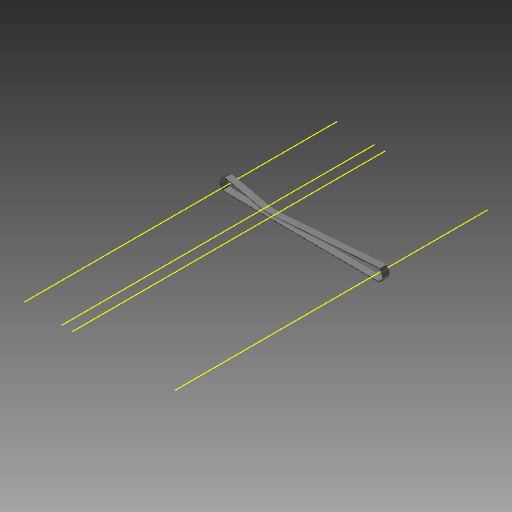
# Autodesk Inventor part: Zahnriemen
Saved by Autodesk Inventor 2019.1 (Build 231200000, 200)
## iProperties
Created: 2018-10-30
Part Number: Zahnriemen
Material: Rubber
Document SubType Name: Modeling
Designer: JochenAlt
Density: 1 g/cm^3
Appearance: Rubber - Black - Version 1.1
CustomPartVersion: 1
Author: JochenAlt
Autodesk Inventor part; units mm, degrees
ref_plane "YZ Plane" through (0, 0, 0) normal (1, 0, 0) x (0, 1, 0)
ref_plane "XZ Plane" through (0, 0, 0) normal (0, 1, 0) x (-1, 0, 0)
ref_plane "XY Plane" through (0, 0, 0) normal (0, 0, 1) x (1, 0, 0)
sketch "Skizzenpfad" plane through (0, 0, 0) normal (0, 0, 1) x (1, 0, 0)
  arc A0 (130.619632, -5.570298) -> (130.240862, 5.554866) centre (130.656885, 0) ccw
  arc A1 (-8.721109, 6.363317) -> (-10.03287, -4.629641) centre (-9.995617, 0.940657) ccw
  arc A2 (24.701763, -1.492183) -> (24.992987, -1.526653) centre (24.999202, -0.226668) ccw
  arc A3 (34.992872, -1.574463) -> (35.096177, -1.570847) centre (34.999088, -0.274478) ccw
  line L0 (35.096177, -1.570847) -> (130.240862, 5.554866)
  line L1 (130.619632, -5.570298) -> (-10.03287, -4.629641)
  line L2 (-8.721109, 6.363317) -> (24.701763, -1.492183)
  line L3 (24.992987, -1.526653) -> (34.992872, -1.574463)
  constraints: 8 end point, 8 point on circle, 4 centre point
ref_plane "Querschnittsebene" through (130.240862, 5.554866, 0) normal (-0.9972072, -0.0746843, 0) x (0, 0, 1)
ref_plane "Arbeitsebene2" through (130.656885, 0, 0) normal (-1, 0, 0) x (0, 0, 1)
ref_plane "Arbeitsebene3" through (-9.995617, 0.940657, 0) normal (0.9456862, -0.3250811, 0) x (0, 0, 1)
sketch "Querschnitt" plane through (130.240862, 5.554866, 0) normal (-0.9972072, -0.0746843, 0) x (0, 0, 1)
  line L0 (-3, 0.3) -> (3, 0.3)
  line L1 (3, 0.3) -> (3, -0.3)
  line L2 (3, -0.3) -> (-3, -0.3)
  line L3 (-3, -0.3) -> (-3, 0.3)
  line L4 (-3, 0) -> (3, 0) construction
  point P0 (0, 0)
  point P1 (0, 0)
  dimension "d0" = 6
  dimension "d4" = 0.3
  dimension "d5" = 0.3
  constraints: 10 end point, 3 midpoint, 2 parallel, 1 coincident, 1 horizontal, 1 perpendicular, 1 other
  measures "d0" distance between parallel lines of L1 L3
  measures "d4" distance between parallel lines of L2 L4
  measures "d5" distance between parallel lines of L4 L0
sweep "Riemen" add profiles "Querschnitt" path "Skizzenpfad" path curves L3 A3 L0 A0 L1 A1 L2 A2
equation "\"d0\" = da_B"
equation "\"d4\" = da_a"
equation "\"d5\" = da_a2"
equation "\"da_B\" = 6"
equation "\"da_pb\" = 2.5"
equation "\"da_L\" = 317.5"
equation "\"da_a\" = 0.3"
equation "\"da_S\" = 1.5"
equation "\"da_Beta\" = 20deg"
equation "\"da_Ht\" = 0.7"
equation "\"da_H\" = 1.3"
equation "\"da_a2\" = 0.3"
body "Solid1"
